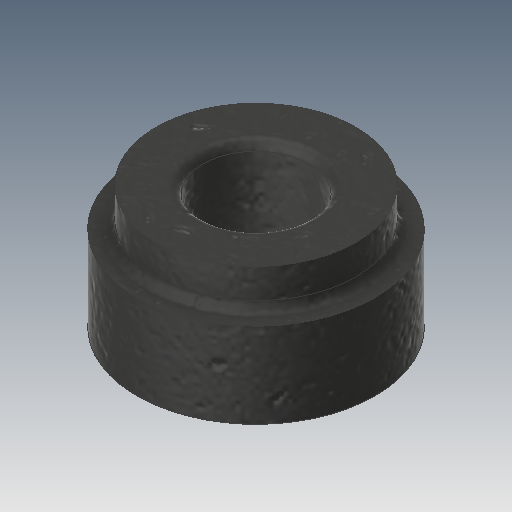
# Autodesk Inventor part: PISTON GUIDE
Saved by Autodesk Inventor 2019 (Build 230136000, 136)
## iProperties
Created: 2023-06-18
Part Number: PISTON GUIDE
Material: Generic
Document SubType Name: Modeling
Designer: Fransic
Density: 1 g/cm^3
Appearance: Fine Textured - Black
Mass: 50.6288 g
Surface Area: 108.132 cm^2
Volume: 50.6288 cm^3
Author: Fransic
Autodesk Inventor part; units mm, degrees
ref_plane "YZ Plane" through (0, 0, 0) normal (1, 0, 0) x (0, 1, 0)
ref_plane "XZ Plane" through (0, 0, 0) normal (0, 1, 0) x (-1, 0, 0)
ref_plane "XY Plane" through (0, 0, 0) normal (0, 0, 1) x (1, 0, 0)
sketch "Sketch1" plane through (0, 0, 0) normal (0, 1, 0) x (-1, 0, 0)
  circle A0 centre (0, 0) radius 28
  dimension "d0" = 56
  constraints: 1 centre point, 1 coincident
  measures "d0" diameter of A0
extrude "Extrusion1" add sketch "Sketch1" along normal blind 20
sketch "Sketch2" plane through (0, 20, 0) normal (0, 1, 0) x (1, 0, 0)
  circle A0 centre (0, 0) radius 23.5
  dimension "d3" = 47
  constraints: 1 centre point, 1 coincident
  measures "d3" diameter of A0
extrude "Extrusion2" add sketch "Sketch2" along normal blind 9
sketch "Sketch3" plane through (0, 29, 0) normal (0, 1, 0) x (1, 0, 0)
  circle A0 centre (0, 0) radius 12.5
  dimension "d6" = 25
  constraints: 1 centre point, 1 coincident
  measures "d6" diameter of A0
extrude "Extrusion3" cut sketch "Sketch3" against normal blind 38
fillet "Fillet1" radius 2 2 edges at (-12.5, 29, 0) (-12.5, 0, 0)
fillet "Fillet2" radius 2 1 edges at (-23.5, 20, 0)
body "Solid1"
